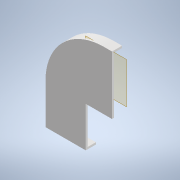
# Autodesk Inventor part: Ring Shooter guide
Saved by Autodesk Inventor 2020 (Build 240168000, 168)
## iProperties
Created: 2020-09-29
Part Number: Ring Shooter guide
Material: Generic
Document SubType Name: Modeling
Designer: jackm
Density: 1 g/cm^3
Appearance: Default
Author: jackm
Autodesk Inventor part; units mm, degrees
ref_plane "YZ Plane" through (0, 0, 0) normal (1, 0, 0) x (0, 1, 0)
ref_plane "XZ Plane" through (0, 0, 0) normal (0, 1, 0) x (-1, 0, 0)
ref_plane "XY Plane" through (0, 0, 0) normal (0, 0, 1) x (1, 0, 0)
ref_plane "Work Plane1" through (0, 0, 0) normal (0, 0, 1) x (1, 0, 0)
sketch "Sketch1" plane through (0, 0, 0) normal (0, 0, 1) x (1, 0, 0)
  circle A0 centre (0, -114.3) radius 4 construction
  line L0 (0, -114.3) -> (-57.15, -114.3) construction
  line L1 (0, -114.3) -> (0, 63.5) construction
  line L2 (25.4, 69.85) -> (0, 69.85)
  arc A1 (0, 69.85) -> (-184.15, -114.3) centre (0, -114.3) ccw
  line L3 (25.4, 69.85) -> (25.4, -114.3)
  line L4 (-184.15, -114.3) -> (-184.15, -241.3)
  line L5 (-184.15, -241.3) -> (-57.15, -241.3)
  line L6 (-57.15, -241.3) -> (-57.15, -119.38)
  line L7 (-57.15, -114.3) -> (-177.8, -114.3) construction
  line L8 (25.4, -114.3) -> (25.4, -119.38)
  line L9 (25.4, -119.38) -> (-57.15, -119.38)
  circle A2 centre (0, -114.3) radius 4
  point P0 (0, 0)
  dimension "d1" = 90
  dimension "d4" = 25.4
  dimension "d5" = 184.15
  dimension "d6" = 127
  dimension "d7" = 127
  dimension "d16" = 5.08
  constraints: 20 end point, 4 perpendicular, 3 coincident, 3 vertical, 2 centre point, 2 point on circle, 1 concentric
  measures "d1" angle of L1 L0
  measures "d4" distance of L2.start L2.end
  measures "d5" radius of A1
  measures "d6" distance of L4.start L4.end
  measures "d7" distance of L4.end L5.end
  measures "d16" distance of L3.end L8.end
extrude "Extrusion1" add sketch "Sketch1" along normal blind 6.35 contours L3 L8 L9 L6 L5 L4 A1 L2 | A2
sketch "Sketch2" plane through (0, 0, 0) normal (0, 0, -1) x (-1, 0, 0)
  arc A0 (184.15, -114.3) -> (0, 69.85) centre (0, -114.3) ccw projected
  line L0 (-25.4, 69.85) -> (0, 69.85) construction
  arc A1 (184.15, -114.3) -> (0, 69.85) centre (0, -114.3) ccw construction
  line L1 (-25.4, -119.38) -> (-25.4, 69.85) construction
  line L2 (0, 69.85) -> (-25.4, 69.85) construction
  line L3 (-25.4, 69.85) -> (-25.4, 63.5) construction
  line L4 (-25.4, 63.5) -> (0, 63.5)
  line L5 (0, 63.5) -> (-25.4, 63.5) construction
  line L6 (-25.4, 69.85) -> (0, 69.85) projected
  line L7 (-25.4, 63.5) -> (-25.4, 69.85)
  line L8 (-25.4, 69.85) -> (0, 69.85)
  arc A2 (177.8, -114.3) -> (0, 63.5) centre (-3.1476, -117.4476) ccw
  line L9 (184.15, -114.3) -> (184.15, -241.3) projected
  line L10 (184.15, -114.3) -> (184.15, -241.3)
  line L11 (184.15, -241.3) -> (57.15, -241.3) projected
  line L12 (184.15, -241.3) -> (57.15, -241.3)
  line L13 (57.15, -241.3) -> (57.15, -234.95)
  line L14 (57.15, -241.3) -> (57.15, -119.38) projected
  line L15 (57.15, -234.95) -> (177.8, -234.95)
  line L16 (177.8, -234.95) -> (177.8, -114.3)
  point P0 (0, 0)
  point P1 (-25.4, -114.3)
  point P2 (57.15, -114.3)
  dimension "d10" = 6.35
  dimension "d11" = 6.35
  dimension "d12" = 180.975
  dimension "d13" = 6.35
  constraints: 22 end point, 4 perpendicular, 4 point on circle, 3 equal length, 2 centre point, 2 point on line, 1 concentric, 1 horizontal, 1 vertical
  measures "d10" distance of L0.start L3.end
  measures "d11" distance of L9.start L16.end
  measures "d12" radius of A2
  measures "d13" distance of L11.end L13.end
extrude "Extrusion2" add sketch "Sketch2" along normal blind 25.4
sketch "Sketch3" plane through (0, 0, 6.35) normal (0, 0, 1) x (1, 0, 0)
  arc A0 (-2.982, -113.9716) -> (-0.8571, -111.4251) centre (0, -114.3) ccw construction
  circle A1 centre (0, -114.3) radius 3
  point P0 (0, 0)
  constraints: 1 centre point, 1 coincident, 1 concentric
extrude "Extrusion3" cut sketch "Sketch3" against normal through all
body "Solid1"
